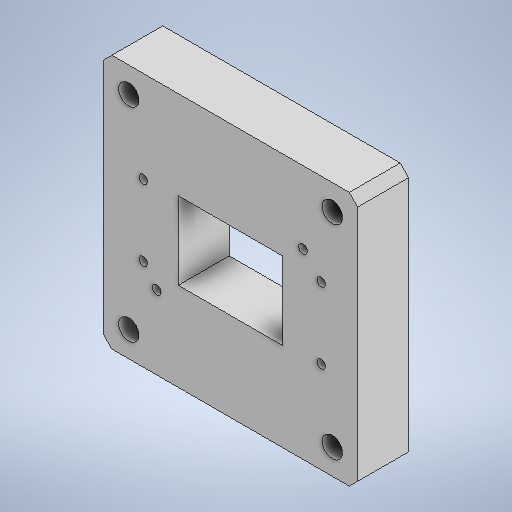
# Autodesk Inventor part: mocowanie_DLP
Saved by Autodesk Inventor 2025.1 (Build 291241000, 241)
## iProperties
Created: 2024-10-24
Part Number: mocowanie_DLP
Material: Ogólny
Document SubType Name: Modeling
Designer: PC
Density: 1 g/cm^3
Appearance: Domyślna
Author: PC
Autodesk Inventor part; units mm, degrees
ref_plane "YZ Plane" through (0, 0, 0) normal (1, 0, 0) x (0, 1, 0)
ref_plane "XZ Plane" through (0, 0, 0) normal (0, 1, 0) x (-1, 0, 0)
ref_plane "XY Plane" through (0, 0, 0) normal (0, 0, 1) x (1, 0, 0)
sketch "Szkic1" plane through (0, 0, 0) normal (0, 0, 1) x (1, 0, 0)
  circle A0 centre (26.725, -10.45) radius 2 projected
  circle A1 centre (26.725, 10.5) radius 2 projected
  circle A2 centre (-25.725, 10.5) radius 2 projected
  circle A3 centre (-25.725, -10.45) radius 2 projected
  arc A4 (8.5, -8.7) -> (12.7, -4.5) centre (8.5, -4.5) ccw projected
  line L0 (8.5, -8.7) -> (-8.5, -8.7) projected
  arc A5 (-12.7, -4.5) -> (-8.5, -8.7) centre (-8.5, -4.5) ccw projected
  line L1 (-12.7, -4.5) -> (-12.7, 4.5) projected
  arc A6 (-8.5, 8.7) -> (-12.7, 4.5) centre (-8.5, 4.5) ccw projected
  line L2 (-8.5, 8.7) -> (8.5, 8.7) projected
  arc A7 (12.7, 4.5) -> (8.5, 8.7) centre (8.5, 4.5) ccw projected
  line L3 (12.7, 4.5) -> (12.7, -4.5) projected
  line L4 (-15.4, -11.43) -> (15.4, -11.43) projected
  line L5 (15.4, -11.43) -> (15.4, 11.43) projected
  line L6 (15.4, 11.43) -> (-15.4, 11.43) projected
  line L7 (-15.4, 11.43) -> (-15.4, -11.43) projected
  arc A8 (-22.3826, -16.8424) -> (-22.8674, -16.3576) centre (-21.775, -15.75) ccw projected
  line L8 (-22.8674, -16.3576) -> (-22.3826, -16.8424) projected
  line L9 (5.5, 4.125) -> (-5.5, 4.125) projected
  line L10 (-5.5, 4.125) -> (-5.5, -4.125) projected
  line L11 (-5.5, -4.125) -> (5.5, -4.125) projected
  line L12 (5.5, -4.125) -> (5.5, 4.125) projected
  circle A9 centre (26.725, -10.45) radius 1.25
  circle A10 centre (26.725, 10.5) radius 1.25
  circle A11 centre (-25.725, 10.5) radius 1.25
  circle A12 centre (-25.725, -10.45) radius 1.25
  circle A13 centre (-21.775, -15.75) radius 1.3
  line L13 (174.975, -22.05) -> (-23.025, -22.05) projected
  line L14 (-35.025, -22.05) -> (20.575, -22.05) projected
  line L15 (-35.025, -22.05) -> (-35.025, -23.55) projected
  line L16 (30, -30) -> (-30, -30) construction
  line L17 (-30, -30) -> (-30, 30) construction
  line L18 (-30, 30) -> (30, 30) construction
  line L19 (30, 30) -> (30, -30) construction
  line L20 (30, -30) -> (-30, 30) construction
  line L21 (-30, -30) -> (30, 30) construction
  line L22 (35, -37.5) -> (-35, -37.5)
  line L23 (-37.5, -35) -> (-37.5, 35)
  line L24 (-35, 37.5) -> (35, 37.5)
  line L25 (37.5, 35) -> (37.5, -35)
  line L26 (37.5, -37.5) -> (-37.5, 37.5) construction
  line L27 (-37.5, -37.5) -> (37.5, 37.5) construction
  circle A14 centre (30, 30) radius 3
  circle A15 centre (30, -30) radius 3
  circle A16 centre (-30, -30) radius 3
  circle A17 centre (-30, 30) radius 3
  line L28 (35, -37.5) -> (37.5, -35)
  line L29 (37.5, 35) -> (35, 37.5)
  line L30 (-37.5, 35) -> (-35, 37.5)
  line L31 (-35, -37.5) -> (-37.5, -35)
  circle A18 centre (21.375, 16.25) radius 1.25 projected
  circle A19 centre (21.375, 16.25) radius 1.3
  line L32 (-15.4, -11.43) -> (-15.4, 11.43) projected
  line L33 (-15.4, 11.43) -> (15.4, 11.43) projected
  line L34 (15.4, 11.43) -> (15.4, -11.43) projected
  line L35 (15.4, -11.43) -> (-15.4, -11.43) projected
  line L36 (-17.907, -13.97) -> (17.907, -13.97) projected
  line L37 (17.907, -13.97) -> (17.907, 13.97) projected
  line L38 (17.907, 13.97) -> (-17.907, 13.97) projected
  line L39 (-17.907, 13.97) -> (-17.907, -13.97) projected
  line L40 (-16, 12) -> (16, 12)
  line L41 (16, 12) -> (16, -12)
  line L42 (16, -12) -> (-16, -12)
  line L43 (-16, -12) -> (-16, 12)
  line L44 (-16, 12) -> (16, -12) construction
  line L45 (16, 12) -> (-16, -12) construction
  point P0 (0, 0)
  dimension "d0" = 2.5
  dimension "d1" = 2.6
  dimension "d3" = 60
  dimension "d4" = 75
  dimension "d5" = 6
  dimension "d6" = 2.5
  dimension "d7" = 2.5
  dimension "d8" = 2.5
  dimension "d9" = 2.5
  dimension "d10" = 2.5
  dimension "d11" = 2.5
  dimension "d12" = 2.5
  dimension "d13" = 2.5
  dimension "d14" = 2.6
  dimension "d21" = 32
  dimension "d22" = 24
  constraints: 44 end point, 10 centre point, 10 coincident, 9 point on line, 6 equal radius, 6 midpoint, 6 parallel, 4 perpendicular, 3 horizontal
  measures "d0" diameter of A9
  measures "d1" diameter of A13
  measures "d3" distance of L17.end L18.end
  measures "d4" distance of L26.end L27.end
  measures "d5" diameter of A14
  measures "d6" distance of L22.start L26.start
  measures "d7" distance of L25.end L26.start
  measures "d8" distance of L25.start L27.end
  measures "d9" distance of L24.end L27.end
  measures "d10" distance of L23.end L26.end
  measures "d11" distance of L24.start L26.end
  measures "d12" distance of L22.end L27.start
  measures "d13" distance of L23.start L27.start
  measures "d14" diameter of A19
  measures "d21" distance of L40.start L40.end
  measures "d22" distance of L40.end L41.end
extrude "Wyciągnięcie proste1" add sketch "Szkic1" along normal blind 15 contours A0 | A1 | A2 | A3 | L22 L31 L23 L30 L24 L29 L25 L28 | L39 L38 L37 L36 | L40 L41 L42 L43
equation "\"d7\" = d6"
equation "\"d8\" = d6"
equation "\"d9\" = d8"
equation "\"d10\" = d6"
equation "\"d11\" = d10"
equation "\"d12\" = d6"
equation "\"d13\" = d12"
